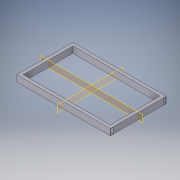
# Autodesk Inventor part: Resized frame
Saved by Autodesk Inventor 2019 (Build 230136000, 136)
## iProperties
Created: 2018-10-13
Part Number: Resized frame
Material: Stainless Steel AISI 440C, Welded
Document SubType Name: Modeling
Designer: olale
Density: 7.8 g/cm^3
Appearance: Weld - Stainless Steel
Mass: 7951.87 g
Surface Area: 6421.86 cm^2
Volume: 1019.47 cm^3
Author: olale
Autodesk Inventor part; units mm, degrees
ref_plane "YZ Plane" through (0, 0, 0) normal (1, 0, 0) x (0, 1, 0)
ref_plane "XZ Plane" through (0, 0, 0) normal (0, 1, 0) x (-1, 0, 0)
ref_plane "XY Plane" through (0, 0, 0) normal (0, 0, 1) x (1, 0, 0)
sketch "Sketch1" plane through (0, 0, 0) normal (1, 0, 0) x (0, 1, 0)
  line L0 (0.0473, 0) -> (50.8473, 0)
  line L1 (50.8473, 0) -> (50.8473, -25.4)
  line L2 (50.8473, -25.4) -> (0.0473, -25.4)
  line L3 (0.0473, -25.4) -> (0.0473, 0)
  line L4 (47.6723, -3.175) -> (3.2223, -3.175)
  line L5 (3.2223, -3.175) -> (3.2223, -22.225)
  line L6 (3.2223, -22.225) -> (47.6723, -22.225)
  line L7 (47.6723, -22.225) -> (47.6723, -3.175)
  dimension "d0" = 25.4
  dimension "d1" = 3.175
  dimension "d2" = 3.175
  dimension "d3" = 3.175
  dimension "d4" = 3.175
  dimension "d5" = 44.45
  constraints: 16 end point, 4 parallel, 2 horizontal, 2 perpendicular
  measures "d0" distance of L0.end L1.end
  measures "d1" distance between parallel lines of L4 L0
  measures "d2" distance between parallel lines of L2 L6
  measures "d3" distance between parallel lines of L1 L7
  measures "d4" distance between parallel lines of L3 L5
  measures "d5" distance between parallel lines of L5 L7
extrude "Extrusion1" add sketch "Sketch1" along normal blind 750.0112
sketch "Sketch2" plane through (0, 0.0473, 0) normal (0, 0, 1) x (1, 0, 0)
  line L0 (0, 0) -> (0, 50.8) projected
  line L1 (0, 0) -> (750.0112, 0) projected
  line L2 (0, 50.8) -> (750.0112, 50.8) projected
  line L3 (0, 0) -> (25.4, 0)
  line L4 (25.4, 0) -> (25.4, 50.8)
  line L5 (25.4, 50.8) -> (0, 50.8)
  line L6 (0, 50.8) -> (0, 0)
  line L7 (3.175, 47.625) -> (22.225, 47.625)
  line L8 (22.225, 47.625) -> (22.225, 3.175)
  line L9 (22.225, 3.175) -> (3.175, 3.175)
  line L10 (3.175, 3.175) -> (3.175, 47.625)
  dimension "d8" = 25.4
  dimension "d9" = 50.8
  dimension "d10" = 3.175
  dimension "d11" = 3.175
  dimension "d12" = 3.175
  dimension "d13" = 3.175
  constraints: 16 end point, 4 parallel, 2 horizontal, 2 perpendicular
  measures "d8" distance of L5.end L4.end
  measures "d9" distance of L4.end L3.end
  measures "d10" distance between parallel lines of L4 L8
  measures "d11" distance between parallel lines of L2 L7
  measures "d12" distance between parallel lines of L1 L9
  measures "d13" distance between parallel lines of L0 L10
extrude "Extrusion2" add sketch "Sketch2" along normal blind 399.2118
ref_plane "Work Plane1" through (375.0056, 0, 0) normal (1, 0, 0) x (0, 0, -1)
mirror "Mirror1" about plane through (375.0056, 0, 0) normal (1, 0, 0) of "Extrusion2"
ref_plane "Work Plane2" through (25.4, 0.0473, 199.6059) normal (0, 0, 1) x (1, 0, 0)
mirror "Mirror2" about plane through (25.4, 0.0473, 199.6059) normal (0, 0, 1) of "Extrusion1"
body "Solid1"
